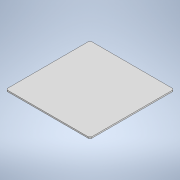
# Autodesk Inventor part: print_platform
Saved by Autodesk Inventor 2020 (Build 240168000, 168)
## iProperties
Created: 2020-01-19
Part Number: print_platform
Material: Generic
Document SubType Name: Modeling
Designer: psrobotics
Density: 1 g/cm^3
Appearance: Default
Author: psrobotics
Autodesk Inventor part; units mm, degrees
ref_plane "YZ Plane" through (0, 0, 0) normal (1, 0, 0) x (0, 1, 0)
ref_plane "XZ Plane" through (0, 0, 0) normal (0, 1, 0) x (-1, 0, 0)
ref_plane "XY Plane" through (0, 0, 0) normal (0, 0, 1) x (1, 0, 0)
sketch "Sketch1" plane through (0, 0, 0) normal (0, 1, 0) x (-1, 0, 0)
  line L0 (62.5, 62.5) -> (62.5, -62.5)
  line L1 (62.5, -62.5) -> (-62.5, -62.5)
  line L2 (-62.5, -62.5) -> (-62.5, 62.5)
  line L3 (-62.5, 62.5) -> (62.5, 62.5)
  line L4 (62.5, 62.5) -> (-62.5, -62.5) construction
  line L5 (62.5, -62.5) -> (-62.5, 62.5) construction
  point P0 (0, 0)
  dimension "d0" = 125
  dimension "d1" = 125
  constraints: 12 end point, 2 midpoint, 2 parallel, 1 perpendicular, 1 vertical
  measures "d0" distance of L0.start L0.end
  measures "d1" distance of L0.end L1.end
extrude "Extrusion1" add sketch "Sketch1" along normal blind 2
chamfer "Chamfer1" distance 2 angle 45 4 edges at (-62.5, 1, 62.5) (62.5, 1, 62.5) (-62.5, 1, -62.5) (62.5, 1, -62.5)
body "Solid1"
